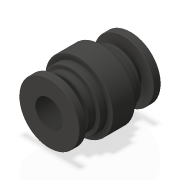
# Autodesk Inventor part: arris_schwingungsdämpfer
Saved by Autodesk Inventor 2016 (Build 200138000, 138)
## iProperties
Created: 2016-04-01
Part Number: arris_schwingungsdämpfer
Material: Gummi, Silikon
Document SubType Name: Modeling
Designer: Stephan
Density: 1.25 g/cm^3
Appearance: Gummi - schwarz
Author: Stephan
Autodesk Inventor part; units mm, degrees
ref_plane "YZ Plane" through (0, 0, 0) normal (1, 0, 0) x (0, 1, 0)
ref_plane "XZ Plane" through (0, 0, 0) normal (0, 1, 0) x (-1, 0, 0)
ref_plane "XY Plane" through (0, 0, 0) normal (0, 0, 1) x (1, 0, 0)
sketch "Skizze1" plane through (0, 0, 0) normal (0, 0, 1) x (1, 0, 0)
  line L0 (0, 10.5) -> (7.75, 10.5)
  line L1 (7.75, 10.5) -> (7.75, 8.6)
  line L2 (7.75, 8.6) -> (4.5, 8.6)
  line L3 (4.5, 8.6) -> (4.5, 6.8)
  line L4 (4.5, 6.8) -> (6.4, 6.8)
  line L5 (6.4, 6.8) -> (6.4, 4.9)
  line L6 (6.4, 4.9) -> (7.4, 4.9)
  line L7 (7.4, 4.9) -> (7.4, 2.9)
  line L8 (7.4, 2.9) -> (8.75, 2.9)
  line L9 (8.75, 2.9) -> (8.75, 0)
  line L10 (8.75, 0) -> (0, 0)
  line L11 (0, 0) -> (0, 10.5)
  line L12 (3.5, 10.5) -> (3.5, 0)
  line L13 (3.5, 4.5) -> (5, 4.5)
  line L14 (5, 4.5) -> (5, 0)
  dimension "d1" = 7
  dimension "d3" = 1.9
  dimension "d4" = 1.8
  dimension "d5" = 1.9
  dimension "d6" = 9
  dimension "d7" = 17.5
  dimension "d8" = 15.5
  dimension "d9" = 12.8
  dimension "d11" = 14.8
  dimension "d12" = 5.8
  dimension "d13" = 6
  dimension "d14" = 10
  dimension "d16" = 13.6
  constraints: 30 end point, 13 perpendicular, 4 point on line, 1 horizontal
  measures "d1" diameter of L12 L11
  measures "d3" distance of L0.end L1.end
  measures "d4" distance of L2.end L3.end
  measures "d5" distance of L4.end L5.end
  measures "d6" diameter of L3 L11
  measures "d7" diameter of L9 L11
  measures "d8" diameter of L1 L11
  measures "d9" diameter of L5 L11
  measures "d11" diameter of L7 L11
  measures "d12" diameter of L8 L10
  measures "d13" distance between parallel lines of L0 L13
  measures "d14" diameter of L14 L11
  measures "d16" diameter of L4 L10
revolve "Umdrehung1" add sketch "Skizze1" angle 360 about axis through (0, 0, 0) along (0, 1, 0) contours L0 L1 L2 L3 L4 L5 L6 L7 L8 L9 L10 L14 L13 L12
mirror "Spiegeln1" about plane through (5, 0, 0) normal (0, -1, 0) of "Umdrehung1"
fillet "Rundung1" radius 0.2 10 edges at (-8.75, 2.9, 0) (-7.4, 4.9, 0) (-6.4, 6.8, 0) (-7.75, 8.6, 0) (-7.75, 10.5, 0) (-8.75, -2.9, 0) (-7.4, -4.9, 0) (-6.4, -6.8, 0) (-7.75, -8.6, 0) (-7.75, -10.5, 0)
